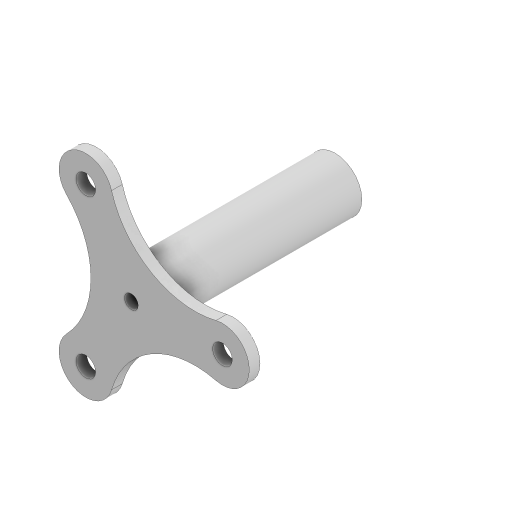
# Autodesk Inventor part: LED Tower
Saved by Autodesk Inventor 2024 (Build 280153000, 153)
## iProperties
Created: 2025-04-26
Part Number: LED Tower
Material: Generic
Document SubType Name: Modeling
Designer: Binara
Density: 1 g/cm^3
Appearance: Default
Author: Binara
Autodesk Inventor part; units mm, degrees
ref_plane "YZ Plane" through (0, 0, 0) normal (1, 0, 0) x (0, 1, 0)
ref_plane "XZ Plane" through (0, 0, 0) normal (0, 1, 0) x (-1, 0, 0)
ref_plane "XY Plane" through (0, 0, 0) normal (0, 0, 1) x (1, 0, 0)
sketch "Block1" plane through (0, 0, 0) normal (0, 0, 1) x (1, 0, 0)
  arc A0 (51.9869, 17.514) -> (51.7404, 14.6963) centre (53.2724, 15.9819) ccw
  arc A1 (68.7213, 13.3186) -> (65.2964, 25.2266) centre (0, 0) ccw
  arc A2 (61.6287, -6.0233) -> (58.811, -6.2699) centre (60.3431, -7.5554) ccw
  arc A3 (61.6287, -6.0233) -> (58.811, -6.2699) centre (60.3431, -7.5554) ccw
  line L0 (61.6287, -6.0233) -> (68.0434, -11.4059)
  line L1 (51.7404, -14.6963) -> (58.811, -6.2699)
  arc A4 (68.7213, -13.3186) -> (68.0434, -11.4059) centre (66.7578, -12.938) ccw
  arc A5 (68.7213, -13.3186) -> (68.0434, -11.4059) centre (66.7578, -12.938) ccw
  arc A6 (51.7404, -14.6963) -> (51.9869, -17.514) centre (53.2724, -15.9819) ccw
  line L2 (62.1452, -26.0379) -> (51.9869, -17.514)
  arc A7 (65.2964, -25.2266) -> (68.7213, -13.3186) centre (0, 0) ccw
  line L3 (68.0434, -11.4059) -> (61.6287, -6.0233)
  arc A8 (62.1452, -26.0379) -> (65.2964, -25.2266) centre (63.4308, -24.5058) ccw
  arc A9 (62.1452, -26.0379) -> (65.2964, -25.2266) centre (63.4308, -24.5058) ccw
  line L4 (36.4337, -56.6797) -> (26.2754, -48.1558)
  line L5 (26.2754, -48.1558) -> (36.4337, -56.6797)
  arc A10 (25.0495, -65.3645) -> (36.1819, -59.9239) centre (0, 0) ccw
  arc A11 (36.1819, -59.9239) -> (36.4337, -56.6797) centre (35.1481, -58.2118) ccw
  arc A12 (36.1819, -59.9239) -> (36.4337, -56.6797) centre (35.1481, -58.2118) ccw
  arc A13 (36.1819, -59.9239) -> (65.2964, -25.2266) centre (0, 0) ccw
  arc A14 (-51.082, -35) -> (-49.082, -33) centre (-51.082, -33) ccw
  line L6 (-49.082, -33) -> (-49.082, -22)
  arc A15 (-66.2353, -22.6471) -> (-61.2046, -33.9706) centre (0, 0) ccw
  line L7 (-49.082, -22) -> (-49.082, -33)
  arc A16 (-51.082, -35) -> (-49.082, -33) centre (-51.082, -33) ccw
  line L8 (-59.4559, -35) -> (-51.082, -35)
  line L9 (-51.082, -35) -> (-59.4559, -35)
  arc A17 (-61.2046, -33.9706) -> (-59.4559, -35) centre (-59.4559, -33) ccw
  arc A18 (-61.2046, -33.9706) -> (-59.4559, -35) centre (-59.4559, -33) ccw
  arc A19 (-49.082, 33) -> (-51.082, 35) centre (-51.082, 33) ccw
  line L10 (-29.1457, 1.2495) -> (-29.1457, -3.1905)
  circle A20 centre (-12.7481, 22.0803) radius 2.75
  arc A21 (25.0495, 65.3645) -> (-61.2046, 33.9706) centre (0, 0) ccw
  circle A22 centre (25.4961, 0) radius 2.75
  line L11 (22.9771, 23.4574) -> (25.8311, 20.0561)
  arc A23 (23.4577, 48.4023) -> (26.2754, 48.1558) centre (24.9898, 49.6879) ccw
  arc A24 (23.4577, 48.4023) -> (26.2754, 48.1558) centre (24.9898, 49.6879) ccw
  arc A25 (16.6335, 59.6465) -> (16.387, 56.8288) centre (17.9191, 58.1144) ccw
  line L12 (16.387, 56.8288) -> (23.4577, 48.4023)
  line L13 (23.4577, 48.4023) -> (16.387, 56.8288)
  arc A26 (-49.082, -22) -> (-51.082, -20) centre (-51.082, -22) ccw
  line L14 (-51.082, -20) -> (-64.3428, -20)
  arc A27 (-64.3428, -20) -> (-66.2353, -22.6471) centre (-64.3428, -22) ccw
  line L15 (-51.082, 20) -> (-64.3428, 20)
  arc A28 (-51.082, 20) -> (-49.082, 22) centre (-51.082, 22) ccw
  arc A29 (-66.2353, 22.6471) -> (-64.3428, 20) centre (-64.3428, 22) ccw
  arc A30 (-66.2353, 22.6471) -> (-64.3428, 20) centre (-64.3428, 22) ccw
  arc A31 (-49.082, -22) -> (-51.082, -20) centre (-51.082, -22) ccw
  line L16 (-64.3428, -20) -> (-51.082, -20)
  arc A32 (-66.2353, 22.6471) -> (-66.2353, -22.6471) centre (0, 0) ccw
  arc A33 (-64.3428, -20) -> (-66.2353, -22.6471) centre (-64.3428, -22) ccw
  line L17 (-64.3428, 20) -> (-51.082, 20)
  line L18 (-49.082, 22) -> (-49.082, 33)
  line L19 (-51.082, 35) -> (-59.4559, 35)
  arc A34 (-59.4559, 35) -> (-61.2046, 33.9706) centre (-59.4559, 33) ccw
  arc A35 (-51.082, 20) -> (-49.082, 22) centre (-51.082, 22) ccw
  line L20 (51.9869, -17.514) -> (62.1452, -26.0379)
  arc A36 (51.7404, -14.6963) -> (51.9869, -17.514) centre (53.2724, -15.9819) ccw
  line L21 (58.811, -6.2699) -> (51.7404, -14.6963)
  line L22 (62.1452, 26.0379) -> (51.9869, 17.514)
  arc A37 (65.2964, 25.2266) -> (62.1452, 26.0379) centre (63.4308, 24.5058) ccw
  arc A38 (65.2964, 25.2266) -> (62.1452, 26.0379) centre (63.4308, 24.5058) ccw
  line L23 (26.2754, 48.1558) -> (36.4337, 56.6797)
  line L24 (36.4337, 56.6797) -> (26.2754, 48.1558)
  arc A39 (36.1819, 59.9239) -> (25.0495, 65.3645) centre (0, 0) ccw
  arc A40 (36.4337, 56.6797) -> (36.1819, 59.9239) centre (35.1481, 58.2118) ccw
  arc A41 (36.4337, 56.6797) -> (36.1819, 59.9239) centre (35.1481, 58.2118) ccw
  arc A42 (65.2964, 25.2266) -> (36.1819, 59.9239) centre (0, 0) ccw
  line L25 (51.9869, 17.514) -> (62.1452, 26.0379)
  arc A43 (-61.2046, 33.9706) -> (-66.2353, 22.6471) centre (0, 0) ccw
  line L26 (-49.082, 33) -> (-49.082, 22)
  arc A44 (-59.4559, 35) -> (-61.2046, 33.9706) centre (-59.4559, 33) ccw
  line L27 (-59.4559, 35) -> (-51.082, 35)
  arc A45 (-49.082, 33) -> (-51.082, 35) centre (-51.082, 33) ccw
  arc A46 (16.387, -56.8288) -> (16.6335, -59.6465) centre (17.9191, -58.1144) ccw
  line L28 (16.6335, -59.6465) -> (23.0483, -65.029)
  arc A47 (23.0483, -65.029) -> (25.0495, -65.3645) centre (24.3338, -63.497) ccw
  arc A48 (26.2754, -48.1558) -> (23.4577, -48.4023) centre (24.9898, -49.6879) ccw
  line L29 (23.4577, -48.4023) -> (16.387, -56.8288)
  arc A49 (-61.2046, -33.9706) -> (25.0495, -65.3645) centre (0, 0) ccw
  arc A50 (16.387, -56.8288) -> (16.6335, -59.6465) centre (17.9191, -58.1144) ccw
  line L30 (23.0483, -65.029) -> (16.6335, -59.6465)
  arc A51 (23.0483, -65.029) -> (25.0495, -65.3645) centre (24.3338, -63.497) ccw
  line L31 (16.387, -56.8288) -> (23.4577, -48.4023)
  arc A52 (26.2754, -48.1558) -> (23.4577, -48.4023) centre (24.9898, -49.6879) ccw
  circle A53 centre (-12.7481, -22.0803) radius 2.75
  arc A54 (16.6335, 59.6465) -> (16.387, 56.8288) centre (17.9191, 58.1144) ccw
  line L32 (23.0483, 65.029) -> (16.6335, 59.6465)
  line L33 (16.6335, 59.6465) -> (23.0483, 65.029)
  arc A55 (25.0495, 65.3645) -> (23.0483, 65.029) centre (24.3338, 63.497) ccw
  arc A56 (25.0495, 65.3645) -> (23.0483, 65.029) centre (24.3338, 63.497) ccw
  arc A57 (58.811, 6.2699) -> (61.6287, 6.0233) centre (60.3431, 7.5554) ccw
  line L34 (61.6287, 6.0233) -> (68.0434, 11.4059)
  arc A58 (68.7213, -13.3186) -> (68.7213, 13.3186) centre (0, 0) ccw
  arc A59 (58.811, 6.2699) -> (61.6287, 6.0233) centre (60.3431, 7.5554) ccw
  line L35 (68.0434, 11.4059) -> (61.6287, 6.0233)
  arc A60 (68.0434, 11.4059) -> (68.7213, 13.3186) centre (66.7578, 12.938) ccw
  arc A61 (68.0434, 11.4059) -> (68.7213, 13.3186) centre (66.7578, 12.938) ccw
  line L36 (51.7404, 14.6963) -> (58.811, 6.2699)
  arc A62 (51.9869, 17.514) -> (51.7404, 14.6963) centre (53.2724, 15.9819) ccw
  line L37 (58.811, 6.2699) -> (51.7404, 14.6963)
  point P0 (9.241, 0.2297)
sketch "Block2" plane through (0, 0, 0) normal (0, 0, 1) x (1, 0, 0)
  line L0 (151.5687, -148.5392) -> (143.1948, -148.5392)
  arc A0 (141.4461, -147.5098) -> (143.1948, -148.5392) centre (143.1948, -146.5392) ccw
  line L1 (254.391, -128.2355) -> (261.4617, -119.809)
  arc A1 (254.391, -128.2355) -> (254.6376, -131.0532) centre (255.9231, -129.5211) ccw
  line L2 (264.7959, -139.5771) -> (254.6376, -131.0532)
  arc A2 (264.7959, -139.5771) -> (267.9471, -138.7657) centre (266.0815, -138.045) ccw
  circle A3 centre (228.1468, -113.5392) radius 2.75
  arc A4 (228.9261, -161.695) -> (226.1084, -161.9415) centre (227.6405, -163.227) ccw
  line L3 (228.9261, -161.695) -> (239.0844, -170.2188)
  arc A5 (238.8326, -173.463) -> (267.9471, -138.7657) centre (202.6507, -113.5392) ccw
  arc A6 (238.8326, -173.463) -> (239.0844, -170.2188) centre (237.7988, -171.7509) ccw
  circle A7 centre (189.9026, -135.6195) radius 2.75
  line L4 (153.5687, -135.5392) -> (153.5687, -146.5392)
  line L5 (158.5687, -148.5392) -> (158.5687, -139.2292)
  line L6 (158.5687, -148.5392) -> (148.1948, -148.5392)
  arc A8 (151.5687, -148.5392) -> (153.5687, -146.5392) centre (151.5687, -146.5392) ccw
  line L7 (174.6507, -139.2292) -> (174.6507, -152.5392)
  line L8 (174.6507, -152.5392) -> (148.1948, -152.5392)
  line L9 (179.6507, -152.5392) -> (179.6507, -139.2292)
  line L10 (148.1948, -152.5392) -> (148.1948, -148.5392)
  arc A9 (143.1948, -78.5392) -> (141.4461, -79.5686) centre (143.1948, -80.5392) ccw
  arc A10 (153.5687, -135.5392) -> (151.5687, -133.5392) centre (151.5687, -135.5392) ccw
  line L11 (138.3079, -133.5392) -> (151.5687, -133.5392)
  arc A11 (138.3079, -133.5392) -> (136.4154, -136.1862) centre (138.3079, -135.5392) ccw
  line L12 (151.5687, -93.5392) -> (138.3079, -93.5392)
  arc A12 (136.4154, -90.8921) -> (136.4154, -136.1862) centre (202.6507, -113.5392) ccw
  arc A13 (136.4154, -90.8921) -> (138.3079, -93.5392) centre (138.3079, -91.5392) ccw
  arc A14 (151.5687, -93.5392) -> (153.5687, -91.5392) centre (151.5687, -91.5392) ccw
  line L13 (143.1948, -78.5392) -> (151.5687, -78.5392)
  arc A15 (153.5687, -80.5392) -> (151.5687, -78.5392) centre (151.5687, -80.5392) ccw
  line L14 (153.5687, -80.5392) -> (153.5687, -91.5392)
  line L15 (158.5687, -139.2292) -> (174.6507, -139.2292)
  arc A16 (254.6376, -96.0252) -> (254.391, -98.8428) centre (255.9231, -97.5572) ccw
  line L16 (254.6376, -96.0252) -> (264.7959, -87.5013)
  arc A17 (267.9471, -88.3126) -> (264.7959, -87.5013) centre (266.0815, -89.0334) ccw
  line L17 (219.9377, -94.8563) -> (222.7917, -98.2575)
  arc A18 (226.1084, -65.1369) -> (228.9261, -65.3834) centre (227.6405, -63.8513) ccw
  arc A19 (267.9471, -88.3126) -> (238.8326, -53.6153) centre (202.6507, -113.5392) ccw
  arc A20 (239.0844, -56.8595) -> (238.8326, -53.6153) centre (237.7988, -55.3274) ccw
  line L18 (239.0844, -56.8595) -> (228.9261, -65.3834)
  line L19 (226.1084, -65.1369) -> (219.0377, -56.7104)
  arc A21 (264.2794, -119.5625) -> (261.4617, -119.809) centre (262.9938, -121.0946) ccw
  line L20 (264.2794, -119.5625) -> (270.6941, -124.9451)
  arc A22 (271.372, -126.8577) -> (270.6941, -124.9451) centre (269.4085, -126.4772) ccw
  arc A23 (261.4617, -107.2693) -> (264.2794, -107.5158) centre (262.9938, -105.9837) ccw
  arc A24 (271.372, -126.8577) -> (271.372, -100.2206) centre (202.6507, -113.5392) ccw
  line L21 (261.4617, -107.2693) -> (254.391, -98.8428)
  line L22 (270.6941, -102.1332) -> (264.2794, -107.5158)
  arc A25 (270.6941, -102.1332) -> (271.372, -100.2206) centre (269.4085, -100.6011) ccw
  circle A26 centre (189.9026, -91.4589) radius 2.75
  line L23 (188.3917, -112.2896) -> (188.3917, -116.7296)
  line L24 (219.2842, -53.8927) -> (225.699, -48.5101)
  arc A27 (227.7002, -48.1746) -> (225.699, -48.5101) centre (226.9845, -50.0422) ccw
  arc A28 (227.7002, -48.1746) -> (141.4461, -79.5686) centre (202.6507, -113.5392) ccw
  arc A29 (219.2842, -53.8927) -> (219.0377, -56.7104) centre (220.5698, -55.4248) ccw
  line L25 (219.2976, -48.6599) -> (221.8687, -51.7241)
  line L26 (213.9219, -58.3922) -> (221.8687, -51.7241)
  line L27 (213.9219, -58.3922) -> (219.9063, -65.5241)
  line L28 (219.9063, -65.5241) -> (207.5867, -75.8614)
  line L29 (213.4899, -70.908) -> (204.9344, -60.712)
  line L30 (199.0312, -65.6654) -> (219.2976, -48.6599)
  line L31 (207.5867, -75.8614) -> (199.0312, -65.6654)
  line L32 (195.201, -68.8793) -> (203.7565, -79.0754)
  arc A30 (141.4461, -147.5098) -> (227.7002, -178.9037) centre (202.6507, -113.5392) ccw
  line L33 (207.5867, -151.2169) -> (199.0312, -161.413)
  line L34 (213.4899, -156.1703) -> (204.9344, -166.3663)
  line L35 (219.9063, -161.5542) -> (207.5867, -151.2169)
  line L36 (213.9219, -168.6861) -> (219.9063, -161.5542)
  arc A31 (219.0377, -170.368) -> (219.2842, -173.1856) centre (220.5698, -171.6535) ccw
  line L37 (199.0312, -161.413) -> (219.2976, -178.4185)
  line L38 (213.9219, -168.6861) -> (221.8687, -175.3543)
  line L39 (219.2976, -178.4185) -> (221.8687, -175.3543)
  line L40 (219.0377, -170.368) -> (226.1084, -161.9415)
  line L41 (225.699, -178.5682) -> (219.2842, -173.1856)
  arc A32 (225.699, -178.5682) -> (227.7002, -178.9037) centre (226.9845, -177.0361) ccw
  line L42 (195.201, -158.199) -> (203.7565, -148.003)
  point P0 (207.2921, -116.2358)
sketch "Sketch1" plane through (0, 0, 0) normal (0, 0, 1) x (1, 0, 0)
  circle A0 centre (188.5512, -95.2219) radius 70
  circle A1 centre (214.0473, -95.2219) radius 2.75
  circle A2 centre (175.8031, -117.3022) radius 2.75
  circle A3 centre (175.8031, -73.1416) radius 2.75
  line L0 (205.1847, -35.5754) -> (211.5995, -30.1928)
  arc A4 (213.6007, -29.8573) -> (211.5995, -30.1928) centre (212.885, -31.7249) ccw
  arc A5 (213.6007, -29.8573) -> (127.3466, -61.2513) centre (188.5512, -95.2219) ccw
  arc A6 (129.0953, -60.2219) -> (127.3466, -61.2513) centre (129.0953, -62.2219) ccw
  line L1 (129.0953, -60.2219) -> (137.4691, -60.2219)
  arc A7 (139.4691, -62.2219) -> (137.4691, -60.2219) centre (137.4691, -62.2219) ccw
  line L2 (139.4691, -62.2219) -> (139.4691, -73.2219)
  arc A8 (137.4691, -75.2219) -> (139.4691, -73.2219) centre (137.4691, -73.2219) ccw
  line L3 (137.4691, -75.2219) -> (124.2084, -75.2219)
  arc A9 (122.3159, -72.5748) -> (124.2084, -75.2219) centre (124.2084, -73.2219) ccw
  arc A10 (122.3159, -72.5748) -> (122.3159, -117.8689) centre (188.5512, -95.2219) ccw
  arc A11 (124.2084, -115.2219) -> (122.3159, -117.8689) centre (124.2084, -117.2219) ccw
  line L4 (124.2084, -115.2219) -> (137.4691, -115.2219)
  arc A12 (139.4691, -117.2219) -> (137.4691, -115.2219) centre (137.4691, -117.2219) ccw
  line L5 (139.4691, -117.2219) -> (139.4691, -128.2219)
  arc A13 (137.4691, -130.2219) -> (139.4691, -128.2219) centre (137.4691, -128.2219) ccw
  line L6 (137.4691, -130.2219) -> (129.0953, -130.2219)
  arc A14 (127.3466, -129.1925) -> (129.0953, -130.2219) centre (129.0953, -128.2219) ccw
  arc A15 (127.3466, -129.1925) -> (213.6007, -160.5864) centre (188.5512, -95.2219) ccw
  arc A16 (211.5995, -160.2509) -> (213.6007, -160.5864) centre (212.885, -158.7188) ccw
  line L7 (211.5995, -160.2509) -> (205.1847, -154.8683)
  arc A17 (204.9382, -152.0507) -> (205.1847, -154.8683) centre (206.4703, -153.3362) ccw
  line L8 (204.9382, -152.0507) -> (212.0089, -143.6242)
  arc A18 (214.8265, -143.3777) -> (212.0089, -143.6242) centre (213.541, -144.9097) ccw
  line L9 (214.8265, -143.3777) -> (224.9849, -151.9015)
  arc A19 (224.7331, -155.1457) -> (224.9849, -151.9015) centre (223.6993, -153.4336) ccw
  arc A20 (224.7331, -155.1457) -> (253.8476, -120.4484) centre (188.5512, -95.2219) ccw
  arc A21 (250.6964, -121.2598) -> (253.8476, -120.4484) centre (251.982, -119.7277) ccw
  line L10 (250.6964, -121.2598) -> (240.5381, -112.7359)
  arc A22 (240.2915, -109.9182) -> (240.5381, -112.7359) centre (241.8236, -111.2038) ccw
  line L11 (240.2915, -109.9182) -> (247.3622, -101.4917)
  arc A23 (250.1799, -101.2452) -> (247.3622, -101.4917) centre (248.8943, -102.7773) ccw
  line L12 (250.1799, -101.2452) -> (256.5946, -106.6278)
  arc A24 (257.2725, -108.5404) -> (256.5946, -106.6278) centre (255.309, -108.1599) ccw
  arc A25 (257.2725, -108.5404) -> (257.2725, -81.9033) centre (188.5512, -95.2219) ccw
  arc A26 (256.5946, -83.8159) -> (257.2725, -81.9033) centre (255.309, -82.2838) ccw
  line L13 (256.5946, -83.8159) -> (250.1799, -89.1985)
  arc A27 (247.3622, -88.952) -> (250.1799, -89.1985) centre (248.8943, -87.6664) ccw
  line L14 (247.3622, -88.952) -> (240.2915, -80.5255)
  arc A28 (240.5381, -77.7079) -> (240.2915, -80.5255) centre (241.8236, -79.2399) ccw
  line L15 (240.5381, -77.7079) -> (250.6964, -69.184)
  arc A29 (253.8476, -69.9953) -> (250.6964, -69.184) centre (251.982, -70.7161) ccw
  arc A30 (253.8476, -69.9953) -> (224.7331, -35.298) centre (188.5512, -95.2219) ccw
  arc A31 (224.9849, -38.5422) -> (224.7331, -35.298) centre (223.6993, -37.0101) ccw
  line L16 (224.9849, -38.5422) -> (214.8265, -47.0661)
  arc A32 (212.0089, -46.8196) -> (214.8265, -47.0661) centre (213.541, -45.534) ccw
  line L17 (212.0089, -46.8196) -> (204.9382, -38.3931)
  arc A33 (205.1847, -35.5754) -> (204.9382, -38.3931) centre (206.4703, -37.1075) ccw
  line L18 (181.1015, -50.562) -> (189.657, -60.7581)
  line L19 (199.3904, -52.5907) -> (190.8349, -42.3947)
  line L20 (193.4872, -57.5441) -> (184.9317, -47.3481)
  line L21 (205.8068, -47.2068) -> (193.4872, -57.5441)
  line L22 (199.8224, -40.0749) -> (205.8068, -47.2068)
  line L23 (199.8224, -40.0749) -> (207.7692, -33.4068)
  line L24 (205.1981, -30.3426) -> (207.7692, -33.4068)
  line L25 (184.9317, -47.3481) -> (205.1981, -30.3426)
  line L26 (160.5512, -120.9119) -> (160.5512, -134.2219)
  line L27 (144.4691, -120.9119) -> (160.5512, -120.9119)
  line L28 (144.4691, -130.2219) -> (144.4691, -120.9119)
  line L29 (144.4691, -130.2219) -> (134.0953, -130.2219)
  line L30 (134.0953, -134.2219) -> (134.0953, -130.2219)
  line L31 (160.5512, -134.2219) -> (134.0953, -134.2219)
  line L32 (199.3904, -137.853) -> (190.8349, -148.049)
  line L33 (193.4872, -132.8996) -> (184.9317, -143.0956)
  line L34 (184.9317, -143.0956) -> (205.1981, -160.1012)
  line L35 (205.1981, -160.1012) -> (207.7692, -157.037)
  line L36 (199.8224, -150.3688) -> (207.7692, -157.037)
  line L37 (199.8224, -150.3688) -> (205.8068, -143.2369)
  line L38 (205.8068, -143.2369) -> (193.4872, -132.8996)
  line L39 (181.1015, -139.8817) -> (189.657, -129.6857)
  line L40 (165.5512, -134.2219) -> (165.5512, -120.9119)
  line L41 (205.8382, -76.539) -> (208.6922, -79.9402)
  line L42 (174.2922, -93.9723) -> (174.2922, -98.4123)
  circle A34 centre (175.8031, -73.1416) radius 7.5
  circle A35 centre (214.0473, -95.2219) radius 7.5
  circle A36 centre (175.8031, -117.3022) radius 7.5
  arc A37 (170.4114, -112.0888) -> (170.4114, -78.355) centre (152.9677, -95.2219) ccw
  circle A38 centre (188.5512, -95.2219) radius 11.3188
  arc A39 (212.2282, -102.4979) -> (183.0139, -119.3648) centre (206.3429, -126.0381) ccw
  arc A40 (183.0139, -71.0789) -> (212.2282, -87.9458) centre (206.3429, -64.4056) ccw
  circle A41 centre (188.5512, -95.2219) radius 1.9291
  point P0 (183.0139, -119.3648)
  point P1 (212.2282, -87.9458)
  point P2 (183.0139, -71.0789)
  dimension "d0" = 15
  dimension "d2" = 15
  dimension "d1" = 15
  dimension "d5" = 360
  constraints: 86 end point, 67 point on circle, 40 centre point, 5 coincident, 1 tangent, 1 vertical, 29 other
  measures "d1" diameter of A35
extrude "Extrusion1" add sketch "Sketch1" along normal blind 3 contours A34 | A34 A40 A38 A37 | A40 A35 A39 A38 | A38 | A38 A39 A36 A37 | A35 | A36
sketch "Sketch2" plane through (0, 0, 0) normal (0, 0, -1) x (-1, 0, 0)
  arc A0 (-183.0139, -119.3648) -> (-212.2282, -102.4979) centre (-206.3429, -126.0381) ccw projected
  arc A1 (-183.0139, -119.3648) -> (-170.4114, -112.0888) centre (-175.8031, -117.3022) ccw projected
  arc A2 (-170.4114, -78.355) -> (-170.4114, -112.0888) centre (-152.9677, -95.2219) ccw projected
  arc A3 (-170.4114, -78.355) -> (-183.0139, -71.0789) centre (-175.8031, -73.1416) ccw projected
  arc A4 (-212.2282, -87.9458) -> (-183.0139, -71.0789) centre (-206.3429, -64.4056) ccw projected
  arc A5 (-212.2282, -87.9458) -> (-212.2282, -102.4979) centre (-214.0473, -95.2219) ccw projected
  circle A6 centre (-214.0473, -95.2219) radius 2.75 projected
  circle A7 centre (-175.8031, -73.1416) radius 2.75 projected
  circle A8 centre (-188.5512, -95.2219) radius 1.9291 projected
  circle A9 centre (-175.8031, -117.3022) radius 2.75 projected
  circle A10 centre (-188.5512, -95.2219) radius 7.5
  point P0 (0, 0)
  dimension "d9" = 15
  constraints: 1 centre point, 1 coincident
  measures "d9" diameter of A10
extrude "Extrusion2" add sketch "Sketch2" along normal blind 54 contours A10
body "Solid1"
